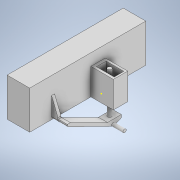
# Autodesk Inventor part: пример подвески 1
Saved by Autodesk Inventor 2020.1 (Build 241239000, 239)
## iProperties
Created: 2021-12-15
Part Number: пример подвески 1
Material: Типовые
Document SubType Name: Modeling
Designer: Ni3na
Density: 1 g/cm^3
Appearance: По умолчанию
Author: Ni3na
Autodesk Inventor part; units mm, degrees
ref_plane "YZ Plane" through (0, 0, 0) normal (1, 0, 0) x (0, 1, 0)
ref_plane "XZ Plane" through (0, 0, 0) normal (0, 1, 0) x (-1, 0, 0)
ref_plane "XY Plane" through (0, 0, 0) normal (0, 0, 1) x (1, 0, 0)
sketch "Эскиз1" plane through (0, 0, 0) normal (1, 0, 0) x (0, 1, 0)
  line L0 (10.9892, 24.817) -> (-5.9609, 24.817)
  line L1 (-5.9609, 24.817) -> (-5.9609, -26.6418)
  line L2 (-5.9609, -26.6418) -> (10.9892, -26.6418)
  line L3 (10.9892, -26.6418) -> (10.9892, 24.817)
  point P0 (0, 0)
  constraints: 8 end point, 2 parallel, 1 horizontal, 1 perpendicular
extrude "Выдавливание1" add sketch "Эскиз1" along normal blind 10
sketch "Эскиз2" plane through (10, 0, 0) normal (1, 0, 0) x (0, 0, -1)
  line L0 (-24.817, -5.9609) -> (26.6418, -5.9609) projected
  line L1 (8.6766, -5.9609) -> (2.3125, -5.9609)
  line L2 (2.3125, -5.9609) -> (2.3125, -4.2236)
  line L3 (2.3125, -4.2236) -> (8.6766, -4.2236)
  line L4 (8.6766, -4.2236) -> (8.6766, -5.9609)
  point P0 (0, 0)
  constraints: 8 end point, 2 parallel, 1 horizontal, 1 perpendicular, 1 point on line
extrude "Выдавливание2" add sketch "Эскиз2" along normal blind 10
sketch "Эскиз3" plane through (10, -4.2236, -2.3125) normal (0, 1, 0) x (1, 0, 0)
  line L0 (9.2453, 5.3703) -> (1.3522, 5.3703)
  line L1 (1.3522, 5.3703) -> (1.3522, 1.0702)
  line L2 (1.3522, 1.0702) -> (9.2453, 1.0702)
  line L3 (9.2453, 1.0702) -> (9.2453, 5.3703)
  point P0 (-10, -2.3125)
  constraints: 8 end point, 2 parallel, 1 horizontal, 1 perpendicular
extrude "Выдавливание3" cut sketch "Эскиз3" against normal blind 10
sketch "Эскиз4" plane through (10, 0, 0) normal (1, 0, 0) x (0, 0, -1)
  circle A0 centre (-14.404, -4.7906) radius 0.7303
  circle A1 centre (5.2437, -14.4688) radius 0.7338
  line L0 (5.2437, -13.7349) -> (-14.0791, -4.1365)
  line L1 (4.6589, -14.9121) -> (-14.7245, -5.4468)
  point P0 (0, 0)
  constraints: 4 end point, 4 point on circle, 2 centre point, 2 tangent
extrude "Выдавливание4" add sketch "Эскиз4" along normal blind 7
sketch "Эскиз5" plane through (10, -4.1365, 14.0791) normal (0, 0.8955929, -0.4448745) x (1, 0, 0)
  line L0 (0, 29.7403) -> (0, -16.3458) projected
  line L1 (0, 0.6764) -> (3.0548, 0.6764)
  line L2 (3.0548, 0.6764) -> (3.0548, 24.6626)
  line L3 (3.0548, 24.6626) -> (0, 24.6626)
  line L4 (0, 24.6626) -> (0, 0.6764)
  point P0 (-10, 10.7689)
  point P1 (0, 24.6626)
  constraints: 8 end point, 2 parallel, 1 horizontal, 1 perpendicular, 1 point on line
extrude "Выдавливание5" cut sketch "Эскиз5" against normal mid plane 10
sketch "Эскиз6" plane through (10, -4.2236, -2.3125) normal (0, 1, 0) x (1, 0, 0)
  circle A0 centre (4.8898, 3.376) radius 0.8761
  point P0 (-10, -2.3125)
  constraints: 1 centre point
extrude "Выдавливание6" add sketch "Эскиз6" along normal mid plane 20
sketch "Эскиз7" plane through (17, 0, 0) normal (1, 0, 0) x (0, 0, -1)
  point P0 (0, 0)
sketch "Эскиз8" plane through (10, -4.2236, -2.3125) normal (0, 1, 0) x (1, 0, 0)
  line L0 (10, 0) -> (10, 6.3641) projected
  line L1 (10, 6.3641) -> (0, 6.3641)
  line L2 (0, 6.3641) -> (0, 0)
  line L3 (0, 0) -> (10, 0)
  line L4 (10, 0) -> (10, 6.3641)
  line L5 (9.2453, 5.3703) -> (1.3522, 5.3703) projected
  line L6 (1.3522, 5.3703) -> (1.3522, 1.0702) projected
  line L7 (9.2453, 5.3703) -> (1.3522, 5.3703)
  line L8 (1.3522, 5.3703) -> (1.3522, 1.0702)
  line L9 (1.3522, 1.0702) -> (9.2453, 1.0702)
  line L10 (9.2453, 1.0702) -> (9.2453, 5.3703)
  point P0 (-10, -2.3125)
  constraints: 16 end point, 4 parallel, 2 horizontal, 2 perpendicular
extrude "Выдавливание7" add sketch "Эскиз8" along normal blind 10
sketch "Эскиз11" plane through (17, 0, 0) normal (1, 0, 0) x (0, 0, -1)
  arc A0 (-14.0791, -4.1365) -> (-14.7245, -5.4468) centre (-14.404, -4.7906) ccw projected
  line L0 (-15.1343, -4.7906) -> (-13.7972, -4.7906)
  line L1 (-13.7972, -4.7906) -> (-13.7972, 3.2916)
  line L2 (-13.7972, 3.2916) -> (-15.1343, 3.2916)
  line L3 (-15.1343, 3.2916) -> (-15.1343, -4.7906)
  point P0 (0, 0)
  constraints: 8 end point, 2 parallel, 1 horizontal, 1 perpendicular, 1 point on circle
extrude "Выдавливание8" add sketch "Эскиз11" against normal blind 10
sketch "Эскиз12" plane through (17, -4.7906, 15.1343) normal (0, 0, 1) x (1, 0, 0)
  line L0 (-7, 0.514) -> (0, 0.514) projected
  line L1 (0, 0.514) -> (-3.9452, 0.514)
  line L2 (-7, 8.0822) -> (-7, 0.514) projected
  line L3 (-3.9452, 0.514) -> (-7, 8.0822)
  line L4 (-7, 8.0822) -> (0, 8.0822)
  line L5 (-3.9452, 0.3531) -> (-7, 0.3531) projected
  line L6 (0, 0.514) -> (0, 8.0822) projected
  line L7 (0, 8.0822) -> (0, 0.514)
  line L8 (0, 0.514) -> (-3.9452, 0.514)
  point P0 (-17, 4.7906)
  constraints: 10 end point, 2 perpendicular, 1 parallel, 1 point on line
extrude "Выдавливание9" cut sketch "Эскиз12" against normal blind 10 contours L3 L4 L6 L0
sketch "Эскиз13" plane through (17, 0, 0) normal (1, 0, 0) x (0, 0, -1)
  line L0 (5.2437, -13.7349) -> (-13.4734, -4.4374) projected
  line L1 (2.6762, -12.4596) -> (8.8225, -12.4596)
  line L2 (8.8225, -12.4596) -> (8.8225, -14.9715)
  line L3 (8.8225, -14.9715) -> (2.6762, -14.9715)
  line L4 (2.6762, -14.9715) -> (2.6762, -12.4596)
  line L5 (-14.1211, -5.7414) -> (4.6589, -14.9121) projected
  line L6 (4.6589, -14.9121) -> (2.6762, -13.9439)
  arc A0 (4.6589, -14.9121) -> (5.2437, -13.7349) centre (5.2437, -14.4688) ccw projected
  line L7 (5.7783, -14.9715) -> (8.8225, -13.7155)
  point P0 (0, 0)
  constraints: 12 end point, 4 point on line, 2 parallel, 1 horizontal, 1 midpoint, 1 perpendicular, 1 point on circle
extrude "Выдавливание10" add sketch "Эскиз13" against normal blind 4 contours L0 L1 L2 L7 A0
sketch "Эскиз14" plane through (13.0548, -4.2766, 15.1343) normal (0, 1, 0) x (1, 0, 0)
  line L0 (0, 1.0132) -> (0, 19.7932) projected
  line L1 (0, 1.9544) -> (-0.2115, 1.9544)
  line L2 (-0.2115, 1.9544) -> (-0.2115, -0.5785)
  line L3 (-0.2115, -0.5785) -> (0, -0.5785)
  line L4 (0, -0.5785) -> (0, 1.9544)
  point P0 (-13.0548, 15.1343)
  constraints: 8 end point, 2 parallel, 1 horizontal, 1 perpendicular, 1 point on line
extrude "Выдавливание11" cut sketch "Эскиз14" along normal mid plane 10
sketch "Эскиз15" plane through (17, 0, 0) normal (1, 0, 0) x (0, 0, -1)
  arc A0 (5.7783, -14.9715) -> (5.2437, -13.7349) centre (5.2437, -14.4688) ccw projected
  circle A1 centre (5.2437, -14.4688) radius 0.7338
  point P0 (0, 0)
  point P1 (5.2437, -13.7349)
  constraints: 1 centre point, 1 coincident
extrude "Выдавливание12" add sketch "Эскиз15" along normal blind 5
